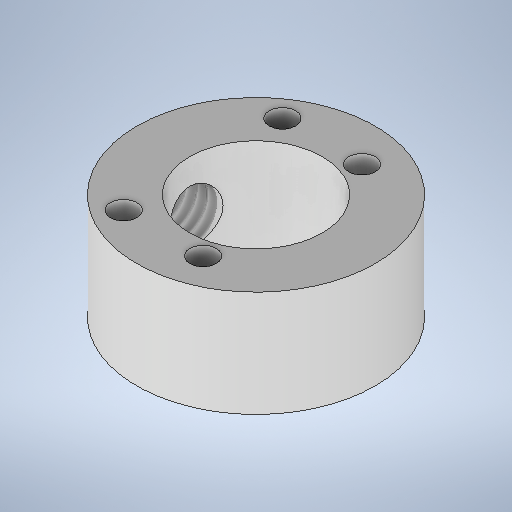
# Autodesk Inventor part: 13
Saved by Autodesk Inventor 2025.1 (Build 291241000, 241)
## iProperties
Created: 2024-09-17
Part Number: 13
Material: Generisch
Document SubType Name: Modeling
Designer: ffogue
Density: 1 g/cm^3
Appearance: Vorgabe
Author: ffogue
Autodesk Inventor part; units mm, degrees
ref_plane "XZ Plane" through (0, 0, 0) normal (0, 1, 0) x (-1, 0, 0)
ref_plane "XY Plane" through (0, 0, 0) normal (0, 0, 1) x (1, 0, 0)
sketch "Sketch1" plane through (0, 0, 0) normal (0, 0, 1) x (1, 0, 0)
  circle A0 centre (0, 0) radius 9
  circle A1 centre (-4, 6) radius 1
  circle A2 centre (2, 6) radius 1
  circle A3 centre (2, -6) radius 1
  circle A4 centre (-4, -6) radius 1
  dimension "d0" = 18
  dimension "d2" = 2
  dimension "d3" = 12
  dimension "d4" = 6
  dimension "d6" = 4
  dimension "d7" = 6
  dimension "d8" = 2
  dimension "d15" = 2
  constraints: 5 centre point, 2 equal radius, 2 horizontal alignment, 2 vertical alignment, 1 coincident
  measures "d0" diameter of A0
  measures "d2" diameter of A4
  measures "d3" distance of A4.centre A1.centre
  measures "d4" vertical distance of point (0, 0) A4.centre
  measures "d6" horizontal distance of point (0, 0) A4.centre
  measures "d7" vertical distance of point (0, 0) A1.centre
  measures "d8" diameter of A1
  measures "d15" horizontal distance of point (0, 0) A3.centre
extrude "Extrusion1" add sketch "Sketch1" along normal blind 8
sketch "Sketch2" plane through (0, 0, 8) normal (0, 0, -1) x (-1, 0, 0)
  circle A0 centre (0, 0) radius 5
  circle A1 centre (-2, 6) radius 1 projected
  dimension "d11" = 10
  constraints: 2 coincident, 1 centre point
  measures "d11" diameter of A0
extrude "Extrusion2" cut sketch "Sketch2" along normal blind 18 contours A0
ref_plane "Work Plane1" through (-9, 0, 0) normal (1, 0, 0) x (0, 1, 0)
sketch "Sketch3" plane through (-9, 0, 0) normal (1, 0, 0) x (0, 1, 0)
  line L0 (9, 8) -> (-9, 8) projected
  line L1 (9, 0) -> (-9, 0) projected
  line L2 (9, 0) -> (9, 8) projected
  point P0 (0, 0)
  point P1 (0, 4)
  point P2 (9, 4)
  point P3 (0, 0)
  constraints: 2 midpoint, 2 vertical alignment, 1 horizontal alignment
hole "Hole1" at (-9, 0, 4) direction (1, 0, 0) diameter 4.134 depth 4.5 thread size "M5x0.8" class "6H" standard "ISO Metric profile"
equation "\"d4\" = 0.5 * d3"
body "Solid1"
